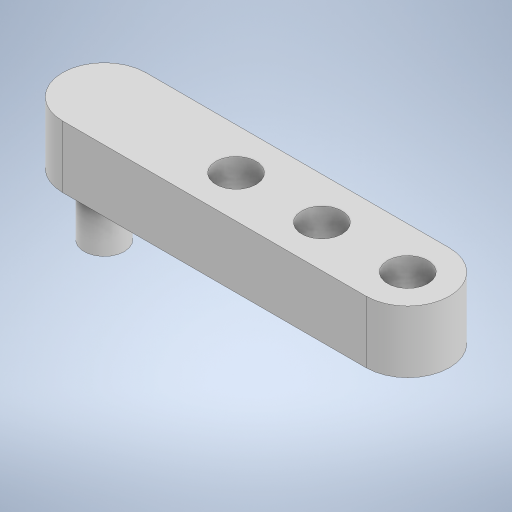
# Autodesk Inventor part: Servo Horn Extension
Saved by Autodesk Inventor 2023 (Build 270158000, 158)
## iProperties
Created: 2023-03-21
Part Number: Servo Horn Extension
Material: Generic
Document SubType Name: Modeling
Designer: 1senadi
Density: 1 g/cm^3
Appearance: Default
Author: 1senadi
Autodesk Inventor part; units mm, degrees
ref_plane "YZ Plane" through (0, 0, 0) normal (1, 0, 0) x (0, 1, 0)
ref_plane "XZ Plane" through (0, 0, 0) normal (0, 1, 0) x (-1, 0, 0)
ref_plane "XY Plane" through (0, 0, 0) normal (0, 0, 1) x (1, 0, 0)
sketch "Sketch1" plane through (0, 0, 0) normal (0, 1, 0) x (-1, 0, 0)
  circle A0 centre (0, 0) radius 0.465
  dimension "d0" = 0.93
  constraints: 1 centre point, 1 coincident
  measures "d0" diameter of A0
extrude "Extrusion1" add sketch "Sketch1" along normal blind 1.43
sketch "Sketch2" plane through (0, 1.43, 0) normal (0, 1, 0) x (1, 0, 0)
  circle A0 centre (0, 0) radius 0.465 projected
  circle A1 centre (0, 0) radius 0.9625
  line L0 (0, 0) -> (7, 0)
  circle A2 centre (7, 0) radius 0.9625
  line L1 (0, -0.9625) -> (7, -0.9625)
  line L2 (0, 0.9625) -> (7, 0.9625)
  circle A3 centre (7, 0) radius 0.465
  circle A4 centre (5.02, 0) radius 0.465
  circle A5 centre (3.04, 0) radius 0.465
  dimension "d3" = 1.925
  dimension "d4" = 7
  dimension "d5" = 1.925
  dimension "d6" = 0.93
  dimension "d9" = 1.98
  constraints: 6 end point, 5 centre point, 4 point on circle, 3 coincident, 2 horizontal, 2 tangent, 1 parallel, 4 other
  measures "d3" diameter of A1
  measures "d4" distance of L0.start L0.end
  measures "d5" diameter of A2
  measures "d6" diameter of A3
  measures "d9" distance of A3.centre A4.centre
extrude "Extrusion2" add sketch "Sketch2" along normal blind 1.43 contours A0 | A1 | A1 L2 A2 L0 A4 A5 | L0 A5 A4 A2 L1 A1 | A2
body "Solid1"
